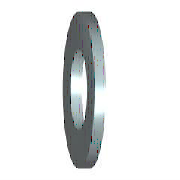
# Autodesk Inventor part: 100009
Saved by Autodesk Inventor 2020.1 (Build 241239000, 239)
## iProperties
Created: 2006-01-26
Part Number: 100009
Material: Steel, Mild
Description: Plain washers - Normal series - Product grade A
Vendor: Autodesk Inc.
Document SubType Name: Modeling
Standard: ISO 7089
Designer: Kevin
Standard Revision: Second edition 2000-06-01
Standards Organization: ISO
Language: en-US
Size Designation: 6 - 140 HV
Categories: <MemberInstance><Categories><Category DisplayName="Fasteners" InternalName="e4da775c-781d-43d5-af7c-5136215cf5a6" Mnemonic="FSTN"><Category DisplayName="Washers" InternalName="337c07a8-832c-4473-9e51-3c1dc967456d" Mnemonic="WSHR"><CategoryParameter DisplayName="Bolt Diameter" InternalName="5ec4e49b-d828-412c-aba4-3e4311d0c7bd" Mnemonic="bltdia"/><CategoryParameter DisplayName="Thickness" InternalName="e5901bd4-d58f-484f-966d-ad4eee01a60f" Mnemonic="wthick"/><Category DisplayName="Plain" InternalName="f89f2849-62ec-45aa-9364-382b706549dc" Mnemonic="PLNWASH"><CategoryParameter DisplayName="Outer Diameter" InternalName="3c824bcc-ed5d-499c-82a4-7ec7de804446" Mnemonic="woutdia"/><CategoryParameter DisplayName="Type" InternalName="5e2e8961-19bf-4ce0-9bfd-17eb8b566124" Mnemonic="type"/></Category></Category></Category></Categories><FamilyTemplate Id="si0008"><FamilyTemplateParameters><FamilyTemplateParameter ObjectType="kUserParameterObject" ValueType="xs:double" Id="1" ObjectReferenceKey="SD1"/><FamilyTemplateParameter ObjectType="kUserParameterObject" ValueType="xs:double" Id="2" ObjectReferenceKey="SD2"/><FamilyTemplateParameter ObjectType="kUserParameterObject" ValueType="xs:double" Id="3" ObjectReferenceKey="SD"/><FamilyTemplateParameter ObjectType="kUserParameterObject" ValueType="xs:double" Id="4" ObjectReferenceKey="NND"/><FamilyTemplateParameter ObjectType="kPropertyObject" ValueType="xs:string" Id="100" ObjectReferenceKey="{32853F0F-3444-11D1-9E93-0060B03C1CA6}" SubObjectId="52"/><FamilyTemplateParameter ObjectType="kPropertyObject" ValueType="xs:string" Id="101" ObjectReferenceKey="{32853F0F-3444-11D1-9E93-0060B03C1CA6}" SubObjectId="49"/><FamilyTemplateParameter ObjectType="kPropertyObject" ValueType="xs:string" Id="102" ObjectReferenceKey="{32853F0F-3444-11D1-9E93-0060B03C1CA6}" SubObjectId="37"/><FamilyTemplateParameter ObjectType="kPropertyObject" ValueType="xs:string" Id="103" ObjectReferenceKey="{32853F0F-3444-11D1-9E93-0060B03C1CA6}" SubObjectId="47"/><FamilyTemplateParameter ObjectType="kPropertyObject" ValueType="xs:string" Id="104" ObjectReferenceKey="{32853F0F-3444-11D1-9E93-0060B03C1CA6}" SubObjectId="48"/><FamilyTemplateParameter ObjectType="kPropertyObject" ValueType="xs:string" Id="105" ObjectReferenceKey="{32853F0F-3444-11D1-9E93-0060B03C1CA6}" SubObjectId="5"/><FamilyTemplateParameter ObjectType="kPropertyObject" ValueType="xs:string" Id="106" ObjectReferenceKey="{32853F0F-3444-11D1-9E93-0060B03C1CA6}" SubObjectId="29"/><FamilyTemplateParameter ObjectType="kPropertyObject" ValueType="xs:string" Id="107" ObjectReferenceKey="{32853F0F-3444-11D1-9E93-0060B03C1CA6}" SubObjectId="20"/><FamilyTemplateParameter ObjectType="kPropertyObject" ValueType="xs:string" Id="108" ObjectReferenceKey="{B9600981-DEE8-4547-8D7C-E525B3A1727A}" SubObjectId="17"/><FamilyTemplateParameter ObjectType="kPropertyObject" ValueType="xs:string" Id="109" ObjectReferenceKey="{B9600981-DEE8-4547-8D7C-E525B3A1727A}" SubObjectId="19"/><FamilyTemplateParameter ObjectType="kPropertyObject" ValueType="xs:string" Id="110" ObjectReferenceKey="{B9600981-DEE8-4547-8D7C-E525B3A1727A}" SubObjectId="21"/><FamilyTemplateParameter ObjectType="kPropertyObject" ValueType="xs:string" Id="111" ObjectReferenceKey="{B9600981-DEE8-4547-8D7C-E525B3A1727A}" SubObjectId="9"/><FamilyTemplateParameter ObjectType="kPartDocumentObject" ValueType="xs:string" Id="112" ObjectReferenceKey="" SubObjectId="DisplayName"/><FamilyTemplateParameter ObjectType="kPartFeatureObject" ValueType="xs:string" Id="400" ObjectReferenceKey="100200001000000092000000000000008000000000000000" SubObjectId="Name"/><FamilyTemplateParameter ObjectType="kPartFeatureObject" ValueType="xs:string" Id="401" ObjectReferenceKey="100200001000000020000000000000008000000000000000" SubObjectId="Name"/><FamilyTemplateParameter ObjectType="kiMateDefinitionObject" ValueType="xs:string" Id="500" ObjectReferenceKey="0401010010000000a38123100c4dbac8fc935889326a8055" SubObjectId="Name"/><FamilyTemplateParameter ObjectType="kiMateDefinitionObject" ValueType="xs:string" Id="501" ObjectReferenceKey="0401010010000000c8546d228445fe9fdf68f69a16664384" SubObjectId="Name"/><FamilyTemplateParameter ObjectType="kiMateDefinitionObject" ValueType="xs:string" Id="502" ObjectReferenceKey="0401010010000000111086d92747f54eb029d991e6675845" SubObjectId="Name"/><FamilyTemplateParameter ObjectType="kiMateDefinitionObject" ValueType="xs:string" Id="503" ObjectReferenceKey="0401010010000000857a3f8e7b4c0ab8488d03be691647b8" SubObjectId="Name"/><FamilyTemplateParameter ObjectType="kiPartTableColumnObject" ValueType="xs:string" Id="504" ObjectReferenceKey="RID"/><FamilyTemplateParameter ObjectType="kiPartTableColumnObject" ValueType="xs:string" Id="505" ObjectReferenceKey="DACOOKIE"/></FamilyTemplateParameters></FamilyTemplate><CategoryParameterMap><ParamToTemplateMap><ParamToTemplate CategoryParameter="//CategoryParameter[@InternalName='316934ee-8fe1-4c7a-9c36-f2d79e1add1a']" TemplateParameter="505"/><ParamToTemplate CategoryParameter="//CategoryParameter[@InternalName='2675968c-4ce5-49e0-a4f5-552d29089031']" TemplateParameter="100"/><ParamToTemplate CategoryParameter="//CategoryParameter[@InternalName='8b46a4cc-9585-4fed-90c3-899f57e09a73']" TemplateParameter="110"/><ParamToTemplate CategoryParameter="//CategoryParameter[@InternalName='818a152a-d3c3-49ca-80ee-df7d91421b8e']" TemplateParameter="107"/><ParamToTemplate CategoryParameter="//CategoryParameter[@InternalName='5ec4e49b-d828-412c-aba4-3e4311d0c7bd']" TemplateParameter="4"/><ParamToTemplate CategoryParameter="//CategoryParameter[@InternalName='016b6077-bfbe-49bd-92c9-d8d59c39c941']" TemplateParameter="105"/><ParamToTemplate CategoryParameter="//CategoryParameter[@InternalName='8e5e0294-fc51-4c8f-b3d7-003dc5ed94f6']" TemplateParameter="504"/><ParamToTemplate CategoryParameter="//CategoryParameter[@InternalName='e5901bd4-d58f-484f-966d-ad4eee01a60f']" TemplateParameter="3"/><ParamToTemplate CategoryParameter="//CategoryParameter[@InternalName='3c824bcc-ed5d-499c-82a4-7ec7de804446']" TemplateParameter="2"/></ParamToTemplateMap></CategoryParameterMap></MemberInstance>
Density: 7.85 g/cm^3
Appearance: Steel
Mass: 1.01645 g
Volume: 0.129484 cm^3
Author: Kevin
Autodesk Inventor part; units mm, degrees
ref_plane "YZ Plane" through (0, 0, 0) normal (1, 0, 0) x (0, 1, 0)
ref_plane "XZ Plane" through (0, 0, 0) normal (0, 1, 0) x (-1, 0, 0)
sketch "Sketch" plane through (0, 0, 0) normal (1, 0, 0) x (0, 1, 0)
  circle A0 centre (0, 0) radius 6
  circle A1 centre (0, 0) radius 3.2
  dimension "d0" = 6.4
  dimension "d1" = 12
  constraints: 2 centre point, 2 coincident
  measures "d0" diameter of A1
  measures "d1" diameter of A0
extrude "Body" add sketch "Sketch" along normal blind 1.6
ref_plane "Work Plane1" through (0, 0, 0) normal (0, 0, 1) x (1, 0, 0)
equation "\"d0\" = SD1"
equation "\"d1\" = SD2"
equation "\"d2\" = SD"
equation "\"SD1\" = 6.4"
equation "\"SD2\" = 12"
equation "\"SD\" = 1.6"
equation "\"NND\" = 6"
body "Solid1"
